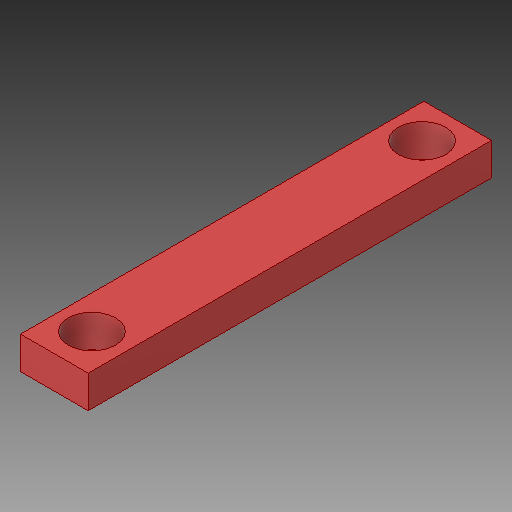
# Autodesk Inventor part: КВ33.044.406 - Прижим ремня
Saved by Autodesk Inventor 2019 (Build 230136000, 136)
## iProperties
Created: 2019-08-20
Part Number: КВ33.044.406 - Прижим ремня
Material: Пластик АБС
Document SubType Name: Modeling
Designer: Петров Иван
Density: 1.06 g/cm^3
Appearance: Гладкий — красный
Mass: 0.330104 g
Surface Area: 4.79334 cm^2
Volume: 0.311419 cm^3
Author: Петров Иван
Autodesk Inventor part; units mm, degrees
ref_plane "YZ Plane" through (0, 0, 0) normal (1, 0, 0) x (0, 1, 0)
ref_plane "XZ Plane" through (0, 0, 0) normal (0, 1, 0) x (-1, 0, 0)
ref_plane "XY Plane" through (0, 0, 0) normal (0, 0, 1) x (1, 0, 0)
sketch "Эскиз2" plane through (0, 0, 0) normal (0, 1, 0) x (-1, 0, 0)
  circle A0 centre (2.5304, -32.2) radius 1.75
  line L0 (0, -30.0054) -> (5, -30.0054)
  line L1 (0, -34.8) -> (0, -30.0054)
  line L2 (5, -34.8) -> (0, -34.8)
  line L3 (5, -30.0054) -> (5, -34.8)
  line L4 (0, -16) -> (5, -16)
  line L5 (0, -24.0054) -> (0, -16)
  line L6 (5, -24.0054) -> (0, -24.0054)
  line L7 (5, -16) -> (5, -24.0054)
  circle A1 centre (2.5304, -7.8054) radius 1.75
  line L8 (5, -10) -> (0, -10)
  line L9 (5, -5) -> (5, -10)
  line L10 (0, -5) -> (5, -5)
  line L11 (0, -10) -> (0, -5)
  line L12 (5, -5) -> (0, -5)
  line L13 (0, -5) -> (0, -34.8)
  line L14 (0, -34.8) -> (5, -34.8)
  line L15 (5, -34.8) -> (5, -5)
  point P0 (0, 0)
  point P1 (5, 0)
  constraints: 32 end point, 2 centre point, 2 parallel, 1 horizontal, 1 perpendicular
extrude "Выдавливание2" add sketch "Эскиз2" along normal blind 2.4
